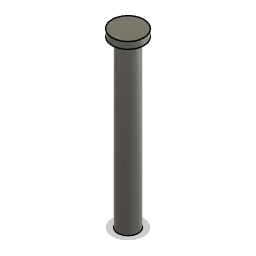
landing gear piston v1 (Autodesk Fusion 360 design; units mm, degrees)
Autodesk Fusion 360 part; units mm, degrees
sketch "Sketch1" plane through (0, 0, 0) normal (0, 0, 1) x (1, 0, 0)
  line L0 (0, 0) -> (0, 380)
  line L1 (0, 380) -> (35, 380)
  line L2 (35, 380) -> (35, 365)
  line L3 (35, 365) -> (22.5, 365)
  line L4 (22.5, 365) -> (22.5, 0)
  line L5 (22.5, 0) -> (0, 0)
  dimension "d2" = 380
  dimension "d3" = 22.5
  dimension "d4" = 35
  dimension "d5" = 15
  constraint coincident L0.start L5.end
  constraint perpendicular L1 L2
  constraint perpendicular L3 L4
  constraint perpendicular L0 L5
  measures "d2" distance of L0.start L0.end
  measures "d3" distance of L4.end L0.start
  measures "d4" distance of L0.end L1.end
  measures "d5" distance of L1.end L2.end
revolve "Revolve1" add sketch "Sketch1" angle 360 about axis through (0, 0, 0) along (0, 1, 0)
